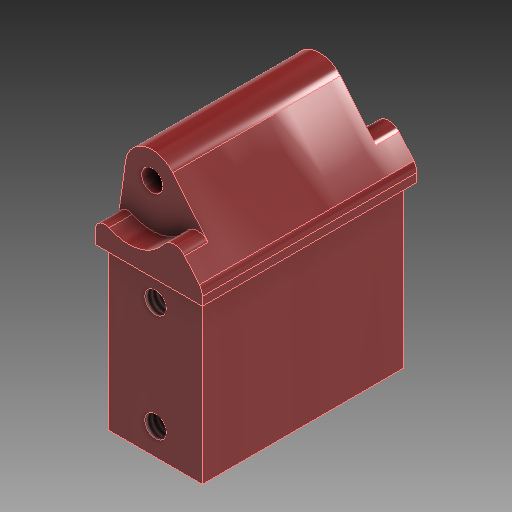
# Autodesk Inventor part: F4C9-200-001 Top Bearing Block
Saved by Autodesk Inventor 2022 (Build 260153000, 153)
## iProperties
ItemSpecifications: {"_id":"606dcdda52f5820009d3f0cd","finish":"543ef1f380da5b0c476373c1","finish_location":null,"material":"5515e170db035c20ce34af9a","process_initialism":null,"quotes":null,"current_quote":null,"quantity_ordered":1,"features":null,"hardware":null,"threading":null,"part_markings":[],"surface_roughness":null,"tolerance":null,"weld_quantity":null,"Notes":"","certifications":[],"part":null,"revision_num":0,"last_history":null,"inspection_requirement_details":{"inspection_requirement":"std","customer_data_sheet":null},"feedback":null}
Created: 2020-08-09
Part Number: F4C9-200-001 Top Bearing Block
Material: Aluminum 6061
Document SubType Name: Modeling
Designer: Cal
Density: 2.7 g/cm^3
Appearance: Reflective - Red
Author: Cal
Autodesk Inventor part; units mm, degrees
ref_plane "YZ Plane" through (0, 0, 0) normal (1, 0, 0) x (0, 1, 0)
ref_plane "XZ Plane" through (0, 0, 0) normal (0, 1, 0) x (-1, 0, 0)
ref_plane "XY Plane" through (0, 0, 0) normal (0, 0, 1) x (1, 0, 0)
sketch "Sketch1" plane through (0, 0, 0) normal (0, 0, 1) x (1, 0, 0)
  line L0 (-12.7, -20.6375) -> (12.7, -20.6375)
  line L1 (12.7, -20.6375) -> (12.7, 20.6375) construction
  line L2 (12.7, 20.6375) -> (-12.7, 20.6375) construction
  line L3 (-12.7, 20.6375) -> (-12.7, -20.6375) construction
  line L4 (-12.7, -20.6375) -> (12.7, 20.6375) construction
  line L5 (12.7, -20.6375) -> (-12.7, 20.6375) construction
  circle A0 centre (0, 11.1125) radius 2.54
  circle A1 centre (0, -1.5875) radius 2.54 construction
  circle A2 centre (0, -14.2875) radius 2.54
  circle A3 centre (-4.7625, 31.75) radius 9.525 construction
  circle A4 centre (-4.7625, 31.75) radius 2.4892
  arc A5 (0.1258, 35.803) -> (-11.0533, 32.6149) centre (-4.7625, 31.75) ccw
  line L6 (-12.7, 20.6375) -> (-11.0533, 32.6149)
  line L7 (12.7, 20.6375) -> (0.1258, 35.803)
  line L8 (-12.7, 20.6375) -> (-11.1125, 20.6375) construction
  line L9 (-11.1125, 20.6375) -> (-11.1125, -20.6375)
  line L10 (11.1125, -20.6375) -> (11.1125, 20.6375)
  line L11 (12.7, 20.6375) -> (11.1125, 20.6375) construction
  line L12 (-12.7, 20.6375) -> (-12.7, 17.4625)
  line L13 (-11.1125, 17.4625) -> (-12.7, 17.4625)
  line L14 (12.7, 20.6375) -> (12.7, 17.4625)
  line L15 (12.7, 17.4625) -> (11.1125, 17.4625)
  point P0 (0, 0)
  point P1 (0, 0)
  dimension "d0" = 25.4
  dimension "d2" = 5.08
  dimension "d3" = 9.525
  dimension "d6" = 12.7
  dimension "d11" = 6.35
  dimension "d12" = 19.05
  dimension "d13" = 4.9784
  dimension "d14" = 11.1125
  dimension "d15" = 4.7625
  dimension "d27" = 1.5875
  dimension "d28" = 1.5875
  dimension "d32" = 3.175
  dimension "d45" = 12.7
  constraints: 32 end point, 8 point on line, 6 centre point, 5 perpendicular, 3 midpoint, 2 horizontal, 2 parallel, 2 point on circle, 2 tangent, 1 coincident, 1 collinear, 1 vertical, 1 vertical alignment, 4 other
  measures "d0" distance of L2.end L1.end
  measures "d2" diameter of A0
  measures "d3" distance from line of A0.centre L2
  measures "d6" distance of A0.centre A1.centre
  measures "d11" distance from line of L0 A2.centre
  measures "d12" diameter of A3
  measures "d13" diameter of A4
  measures "d14" distance from line of L2 A3.centre
  measures "d15" horizontal distance of A0.centre A3.centre
  measures "d27" distance between parallel lines of L3 L9
  measures "d28" distance between parallel lines of L1 L10
  measures "d32" distance between parallel lines of L13 L2
  measures "d45" diameter of A5
extrude "Extrusion1" add sketch "Sketch1" along normal mid plane 50.8
sketch "Sketch3" plane through (-11.1125, -20.6375, 25.4) normal (-1, 0, 0) x (0, 0, 1)
  line L0 (-50.8, 0) -> (0, 0) projected
  line L1 (0, 38.1) -> (0, 0) projected
  line L2 (-50.8, 0) -> (-50.8, 38.1) projected
  line L3 (-49.2125, 41.275) -> (-1.5875, 41.275)
  line L4 (-1.5875, 41.275) -> (-1.5875, 0)
  line L5 (-1.5875, 0) -> (-49.2125, 0)
  line L6 (-49.2125, 0) -> (-49.2125, 41.275)
  line L7 (-49.2125, 41.275) -> (-1.5875, 0) construction
  line L8 (-1.5875, 41.275) -> (-49.2125, 0) construction
  line L9 (-50.8, 38.1) -> (0, 38.1) projected
  point P0 (-25.4, 20.6375)
  point P1 (-49.2125, 38.1)
  point P2 (-1.5875, 38.1)
  dimension "d29" = 1.5875
  constraints: 12 end point, 2 midpoint, 2 parallel, 1 horizontal, 1 perpendicular, 1 point on line
  measures "d29" distance between parallel lines of L1 L4
extrude "Extrusion3" cut sketch "Sketch3" against normal through all contours L2 L9 L6 L0 | L4 L9 L1 L0
sketch "Sketch2" plane through (0, 0, 25.4) normal (0, 0, 1) x (1, 0, 0)
  circle A0 centre (-4.7625, 31.75) radius 2.4892 projected
  circle A1 centre (-4.7625, 31.75) radius 10.3188
  point P0 (0, 0)
  dimension "d19" = 20.6375
  constraints: 1 centre point, 1 coincident
  measures "d19" diameter of A1
extrude "Extrusion2" cut sketch "Sketch2" against normal blind 5.5563
mirror "Mirror1" about plane through (0, 0, 0) normal (0, 0, 1) of "Extrusion2"
fillet "Fillet1" radius 3.175 3 edges at (5.3172, 29.5418, 22.6219) (5.3172, 29.5418, -22.6219) (12.7, 20.6375, 0)
fillet "Fillet1" radius 2.286 2 edges at (-12.1611, 24.5572, -22.6219) (-12.1611, 24.5572, 22.6219)
thread "Thread1" size "1/4-20 UNC" class "2B" standard "ANSI Unified Screw Threads" length 19.05
thread "Thread2" size "1/4-20 UNC" class "2B" standard "ANSI Unified Screw Threads" length 19.05
thread "Thread3" size "1/4-20 UNC" class "2B" standard "ANSI Unified Screw Threads" length 19.05
thread "Thread4" size "1/4-20 UNC" class "2B" standard "ANSI Unified Screw Threads" length 19.05
sketch "Sketch4" plane through (-11.1125, -20.6375, -23.8125) normal (0, -1, 0) x (1, 0, 0)
  line L0 (0, 0) -> (22.225, 0) projected
  line L1 (22.225, 0) -> (22.225, 47.625) projected
  line L2 (22.225, 47.625) -> (0, 47.625) projected
  line L3 (0, 0) -> (0, 47.625) projected
  line L4 (19.05, 41.275) -> (3.175, 41.275)
  line L5 (3.175, 41.275) -> (3.175, 6.35)
  line L6 (3.175, 6.35) -> (19.05, 6.35)
  line L7 (19.05, 6.35) -> (19.05, 41.275)
  point P0 (11.1125, 23.8125)
  dimension "d37" = 3.175
  dimension "d38" = 3.175
  dimension "d39" = 6.35
  dimension "d40" = 6.35
  constraints: 8 end point, 2 parallel, 1 horizontal, 1 perpendicular
  measures "d37" distance between parallel lines of L1 L7
  measures "d38" distance between parallel lines of L3 L5
  measures "d39" distance between parallel lines of L0 L6
  measures "d40" distance between parallel lines of L2 L4
extrude "Extrusion4" cut sketch "Sketch4" against normal up to surface (38.1 mm away) contours L7 L6 L5 L4
fillet "Fillet2" radius 3.175 4 edges at (-7.9375, -1.5875, 17.4625) (7.9375, -1.5875, 17.4625) (7.9375, -1.5875, -17.4625) (-7.9375, -1.5875, -17.4625)
equation "\"d28\" = d27"
equation "\"d38\" = d37"
equation "\"d40\" = d39"
body "Solid1"
